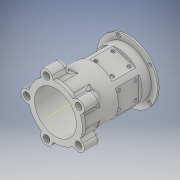
# Autodesk Inventor part: outer
Saved by Autodesk Inventor 2018 (Build 220112000, 112)
## iProperties
Created: 2021-03-13
Part Number: outer
Material: Generic
Document SubType Name: Modeling
Designer: Jyoti Soni
Density: 1 g/cm^3
Appearance: Default
Author: Jyoti Soni
Autodesk Inventor part; units mm, degrees
ref_plane "YZ Plane" through (0, 0, 0) normal (1, 0, 0) x (0, 1, 0)
ref_plane "XZ Plane" through (0, 0, 0) normal (0, 1, 0) x (-1, 0, 0)
ref_plane "XY Plane" through (0, 0, 0) normal (0, 0, 1) x (1, 0, 0)
sketch "Sketch1" plane through (0, 0, 0) normal (0, 0, 1) x (1, 0, 0)
  circle A0 centre (0, 0) radius 62
  circle A1 centre (0, 0) radius 72
  dimension "d0" = 124
  dimension "d1" = 144
  constraints: 2 centre point, 2 coincident
  measures "d0" diameter of A0
  measures "d1" diameter of A1
extrude "Extrusion1" add sketch "Sketch1" against normal blind 217.5
sketch "Sketch2" plane through (0, 0, 0) normal (0, 0, 1) x (1, 0, 0)
  circle A0 centre (0, 0) radius 72 projected
  circle A1 centre (0, 0) radius 80
  dimension "d4" = 160
  constraints: 1 centre point, 1 coincident
  measures "d4" diameter of A1
extrude "Extrusion2" add sketch "Sketch2" against normal blind 10
sketch "Sketch3" plane through (0, 0, -217.5) normal (0, 0, -1) x (-1, 0, 0)
  circle A0 centre (0, 0) radius 72 projected
  circle A1 centre (0, 0) radius 90
  dimension "d7" = 180
  constraints: 1 centre point, 1 coincident
  measures "d7" diameter of A1
extrude "Extrusion3" add sketch "Sketch3" against normal blind 5
sketch "Sketch6" plane through (0, 0, 0) normal (0, 0, 1) x (1, 0, 0)
  circle A0 centre (0, 0) radius 72 construction
  line L0 (0, 0) -> (102.496834, -74.468309) construction
  line L1 (0, 0) -> (124.179406, 0) construction
  circle A1 centre (68.766445, -49.961746) radius 10
  arc A2 (61.096266, -65.691284) -> (81.355908, -37.806278) centre (68.766445, -49.961746) ccw
  line L2 (81.355908, -37.806278) -> (67.920594, -23.891273)
  line L3 (43.710569, -57.213514) -> (61.096266, -65.691284)
  arc A3 (43.710569, -57.213514) -> (67.920594, -23.891273) centre (0, 0) ccw
  dimension "d11" = 36
  dimension "d12" = 20
  dimension "d13" = 35
  dimension "d14" = 85
  constraints: 8 end point, 6 point on circle, 3 centre point, 2 tangent, 1 coincident, 1 horizontal, 1 point on line, 1 other
  measures "d11" angle of L1 L0
  measures "d12" diameter of A1
  measures "d13" diameter of A2
  measures "d14" distance of A1.centre point (0, 0)
extrude "Extrusion4" add sketch "Sketch6" against normal blind 50
sketch "Sketch7" plane through (0, 0, -50) normal (0, 0, -1) x (-1, 0, 0)
  circle A0 centre (-68.766445, -49.961746) radius 10
  arc A1 (-43.710569, -57.213514) -> (-67.920594, -23.891273) centre (0, 0) ccw
  point P0 (-54.724077, -46.789693)
  point P1 (-61.410312, -37.58688)
  constraints: 1 other
extrude "Extrusion5" add sketch "Sketch7" against normal blind 5
fillet "Fillet1" radius 12 3 edges at (58.2492, -42.3205, -50) (67.9206, -23.8913, -30) (43.7106, -57.2135, -30)
fillet "Fillet2" radius 12 7 edges at (74.8853, -31.1046, -50.3586) (79.2193, -35.5934, -50) (82.9242, -60.248, -50) (58.3314, -64.3431, -50) (52.7231, -61.6083, -50.3586) (43.506, -59.1444, -56.3332) (69.6938, -23.0999, -56.3333)
pattern_circular "Circular Pattern1" count 5 over 360 about axis through (0, 0, 0) along (0, 0, -1) of "Fillet2", "Fillet1", "Extrusion5", "Extrusion4", "Extrusion2", "Extrusion1"
sketch "Sketch8" plane through (0, 0, 0) normal (0, 0, 1) x (1, 0, 0)
  arc A0 (-16.605579, 78.257618) -> (-32.564478, 73.072257) centre (-26.266445, 80.839804) ccw construction
  circle A1 centre (-26.266445, 80.839804) radius 10
  point P0 (0, 0)
  constraints: 1 centre point, 1 coincident, 1 concentric
extrude "Extrusion6" cut sketch "Sketch8" against normal blind 40
pattern_circular "Circular Pattern2" count 5 over 360 about axis through (0, 0, 0) along (0, 0, -1) of "Extrusion6"
sketch "Sketch9" plane through (0, 0, -217.5) normal (0, 0, -1) x (-1, 0, 0)
  circle A0 centre (0, 0) radius 82.5 construction
  circle A1 centre (82.5, 0) radius 6
  dimension "d30" = 165
  dimension "d31" = 12
  constraints: 1 centre point, 1 coincident, 1 horizontal alignment, 2 other
  measures "d31" diameter of A1
extrude "Extrusion7" cut sketch "Sketch9" against normal blind 10
pattern_circular "Circular Pattern3" count 5 over 360 about axis through (0, 0, 0) along (0, 0, -1) of "Extrusion7"
ref_plane "Work Plane1" through (0, 0, -150) normal (0, 0, 1) x (1, 0, 0)
sketch "Sketch10" plane through (0, 0, -150) normal (0, 0, 1) x (1, 0, 0)
  circle A0 centre (0, 0) radius 62 construction
  circle A1 centre (0, 0) radius 72 construction
  arc A2 (69.799283, 17.665222) -> (38.36979, 60.924209) centre (0, 0) ccw construction
  arc A3 (69.799283, -17.665222) -> (69.799283, 17.665222) centre (0, 0) ccw construction
  arc A4 (38.36979, -60.924209) -> (69.799283, -17.665222) centre (0, 0) ccw construction
  arc A5 (4.76854, -71.841917) -> (38.36979, -60.924209) centre (0, 0) ccw construction
  arc A6 (-46.085449, -55.318454) -> (4.76854, -71.841917) centre (0, 0) ccw construction
  arc A7 (-66.852163, -26.735524) -> (-46.085449, -55.318454) centre (0, 0) ccw construction
  arc A8 (-66.852163, 26.735524) -> (-66.852163, -26.735524) centre (0, 0) ccw construction
  arc A9 (-46.085449, 55.318454) -> (-66.852163, 26.735524) centre (0, 0) ccw construction
  arc A10 (4.76854, 71.841917) -> (-46.085449, 55.318454) centre (0, 0) ccw construction
  arc A11 (38.36979, 60.924209) -> (4.76854, 71.841917) centre (0, 0) ccw construction
  circle A12 centre (-26.266445, 80.839804) radius 10 construction
  circle A13 centre (68.766445, 49.961746) radius 10 construction
  line L0 (0, 0) -> (-26.266445, 80.839804) construction
  line L1 (0, 0) -> (68.766445, 49.961746) construction
  line L2 (-23.483981, 73.346797) -> (62.111105, 45.535268)
  line L3 (0, 0) -> (33.239809, 102.301612) construction
  line L4 (-23.483981, 73.346797) -> (-18.189189, 89.642493)
  line L5 (62.111105, 45.535268) -> (67.405898, 61.830963)
  line L6 (-18.189189, 89.642493) -> (67.405898, 61.830963)
  dimension "d38" = 36
  dimension "d39" = 45
  dimension "d40" = 45
  dimension "d43" = 62.5
  constraints: 14 end point, 3 parallel
  measures "d38" angle of L3 L0
  measures "d39" distance between parallel lines of L3 L4
  measures "d40" distance from line of L5.end L3
  measures "d43" distance from line of point (0, 0) L2
extrude "Extrusion8" cut sketch "Sketch10" along normal mid plane 70
pattern_circular "Circular Pattern4" count 5 over 360 about axis through (0, 0, 0) along (0, 0, -1) of "Extrusion8"
sketch "Sketch12" plane through (62.5, -35.745629, -185) normal (1, 0, 0) x (0, 0, -1)
  line L0 (-70, 71.491258) -> (0, 71.491258) construction
  line L1 (-35, 71.491258) -> (-35, -89.973642) construction
  line L2 (-70, 71.491258) -> (-70, 0) construction
  line L3 (-70, 71.491258) -> (-70, 0) construction
  line L4 (-70, 35.745629) -> (192.851007, 35.745629) construction
  line L5 (-60, 10.745629) -> (-10, 10.745629) construction
  line L6 (-10, 10.745629) -> (-10, 60.745629) construction
  line L7 (-10, 60.745629) -> (-60, 60.745629) construction
  line L8 (-60, 60.745629) -> (-60, 10.745629) construction
  line L9 (-60, 10.745629) -> (-10, 60.745629) construction
  line L10 (-10, 10.745629) -> (-60, 60.745629) construction
  circle A0 centre (-60, 60.745629) radius 5
  circle A1 centre (-10, 60.745629) radius 5
  circle A2 centre (-10, 10.745629) radius 5
  circle A3 centre (-60, 10.745629) radius 5
  point P0 (-185, 35.745629)
  point P1 (-35, 35.745629)
  dimension "d49" = 50
  dimension "d50" = 50
  dimension "d51" = 10
  constraints: 16 end point, 4 centre point, 4 coincident, 4 midpoint, 3 equal radius, 2 horizontal, 2 parallel, 2 point on line, 1 perpendicular, 1 vertical
  measures "d49" distance of L6.end L7.end
  measures "d50" distance of L5.end L6.end
  measures "d51" diameter of A0
extrude "Extrusion9" cut sketch "Sketch12" against normal blind 20
pattern_circular "Circular Pattern5" count 5 over 360 about axis through (0, 0, 0) along (0, 0, -1) of "Extrusion9"
body "Solid1"
